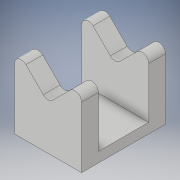
# Autodesk Inventor part: CapillaryHolder
Saved by Autodesk Inventor 2019 (Build 230136000, 136)
## iProperties
Created: 2019-07-22
Part Number: CapillaryHolder
Material: Generic
Document SubType Name: Modeling
Designer: aorfi
Density: 1 g/cm^3
Appearance: Default
Author: aorfi
Autodesk Inventor part; units mm, degrees
ref_plane "YZ Plane" through (0, 0, 0) normal (1, 0, 0) x (0, 1, 0)
ref_plane "XZ Plane" through (0, 0, 0) normal (0, 1, 0) x (-1, 0, 0)
ref_plane "XY Plane" through (0, 0, 0) normal (0, 0, 1) x (1, 0, 0)
sketch "Sketch1" plane through (0, 0, 0) normal (0, 1, 0) x (-1, 0, 0)
  line L0 (-10, 12.5) -> (10, 12.5)
  line L1 (10, 12.5) -> (10, -12.5)
  line L2 (10, -12.5) -> (-10, -12.5)
  line L3 (-10, -12.5) -> (-10, 12.5)
  line L4 (-10, 12.5) -> (10, -12.5) construction
  line L5 (10, 12.5) -> (-10, -12.5) construction
  point P0 (0, 0)
  dimension "d0" = 25
  dimension "d1" = 20
  constraints: 12 end point, 2 midpoint, 2 parallel, 1 horizontal, 1 perpendicular
  measures "d0" distance of L0.end L1.end
  measures "d1" distance of L0.start L0.end
extrude "Extrusion1" add sketch "Sketch1" along normal blind 3
sketch "Sketch2" plane through (0, 3, 0) normal (0, 1, 0) x (1, 0, 0)
  line L0 (-10, 12.5) -> (-10, -12.5) projected
  line L1 (-10, 12.5) -> (10, 12.5)
  line L2 (10, 12.5) -> (10, 7.5)
  line L3 (10, 7.5) -> (-10, 7.5)
  line L4 (-10, 7.5) -> (-10, 12.5)
  line L5 (10, 12.5) -> (-10, 12.5) projected
  line L6 (10, -12.5) -> (10, 12.5) projected
  line L7 (-10, 0) -> (10, 0) construction
  line L8 (-10, -12.5) -> (10, -12.5)
  line L9 (10, -12.5) -> (10, -7.5)
  line L10 (10, -7.5) -> (-10, -7.5)
  line L11 (-10, -7.5) -> (-10, -12.5)
  line L12 (10, -12.5) -> (-10, -12.5)
  point P0 (0, 0)
  dimension "d4" = 5
  constraints: 20 end point, 6 symmetric about line, 2 collinear, 2 midpoint, 2 parallel, 1 horizontal, 1 perpendicular, 1 point on line
  measures "d4" distance between parallel lines of L1 L3
extrude "Extrusion2" add sketch "Sketch2" along normal blind 20 contours L1 L2 L3 L0 | L10 L6 L8 L0
sketch "Sketch3" plane through (10, 0, -12.5) normal (0, 0, -1) x (-1, 0, 0)
  line L0 (20, 23) -> (0, 23) projected
  line L1 (0, 23) -> (10, 13)
  line L2 (10, 13) -> (20, 23)
  line L3 (20, 0) -> (0, 0) projected
  point P0 (10, 0)
  point P1 (10, 0)
  constraints: 4 end point, 1 midpoint, 1 perpendicular, 1 vertical alignment
extrude "Extrusion3" cut sketch "Sketch3" against normal through all
fillet "Fillet1" radius 2 6 edges at (0, 13, -10) (0, 13, 10) (10, 23, -10) (-10, 23, -10) (-10, 23, 10) (10, 23, 10)
sketch "Sketch4" plane through (0, 3, 0) normal (0, 1, 0) x (1, 0, 0)
  point P0 (0, 0)
body "Solid1"
